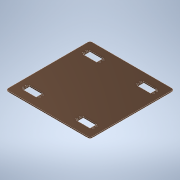
# Autodesk Inventor part: RobotBase
Saved by Autodesk Inventor 2022.3 (Build 263350000, 350)
## iProperties
Created: 2022-04-28
Part Number: RobotBase
Material: Bronze, Cast
Document SubType Name: Modeling
Designer: Robert Nies
Density: 8.87 g/cm^3
Appearance: Bronze - Satin
Author: Robert Nies
Autodesk Inventor part; units mm, degrees
ref_plane "YZ Plane" through (0, 0, 0) normal (1, 0, 0) x (0, 1, 0)
ref_plane "XZ Plane" through (0, 0, 0) normal (0, 1, 0) x (-1, 0, 0)
ref_plane "XY Plane" through (0, 0, 0) normal (0, 0, 1) x (1, 0, 0)
sketch "Sketch1" plane through (0, 0, 0) normal (0, 1, 0) x (-1, 0, 0)
  line L0 (0, 0) -> (-254, 0)
  line L1 (-254, 0) -> (-254, -254)
  line L2 (-254, -254) -> (0, -254)
  line L3 (0, -254) -> (0, 0)
  dimension "d0" = 254
  dimension "d1" = 254
  constraints: 8 end point, 2 parallel, 1 horizontal, 1 perpendicular
  measures "d0" distance of L2.end L1.end
  measures "d1" distance of L1.end L0.end
extrude "Extrusion1" add sketch "Sketch1" along normal blind 3.175
fillet "Fillet1" radius 6.35 4 edges at (0, 1.5875, 0) (254, 1.5875, 0) (254, 1.5875, -254) (0, 1.5875, -254)
sketch "Sketch2" plane through (0, 3.175, 0) normal (0, 1, 0) x (1, 0, 0)
  line L0 (247.65, 254) -> (6.35, 254) projected
  line L1 (0, 247.65) -> (0, 6.35) projected
  line L2 (25.4, 45.72) -> (66.04, 45.72)
  line L3 (66.04, 45.72) -> (66.04, 25.4)
  line L4 (66.04, 25.4) -> (25.4, 25.4)
  line L5 (25.4, 25.4) -> (25.4, 45.72)
  line L6 (254, 6.35) -> (254, 247.65) projected
  line L7 (6.35, 0) -> (247.65, 0) projected
  circle A0 centre (20.955, 30.635) radius 2.1828
  circle A1 centre (20.955, 40.485) radius 2.1828
  circle A2 centre (70.485, 40.485) radius 2.1828
  circle A3 centre (70.485, 30.635) radius 2.1828
  line L8 (25.4, 228.6) -> (66.04, 228.6)
  line L9 (66.04, 228.6) -> (66.04, 208.28)
  line L10 (66.04, 208.28) -> (25.4, 208.28)
  line L11 (25.4, 208.28) -> (25.4, 228.6)
  circle A4 centre (20.955, 213.515) radius 2.1828
  circle A5 centre (20.955, 223.365) radius 2.1828
  circle A6 centre (70.485, 223.365) radius 2.1828
  circle A7 centre (70.485, 213.515) radius 2.1828
  circle A8 centre (233.045, 223.365) radius 2.1828
  circle A9 centre (233.045, 213.515) radius 2.1828
  line L12 (228.6, 228.6) -> (228.6, 208.28)
  line L13 (187.96, 228.6) -> (228.6, 228.6)
  line L14 (228.6, 208.28) -> (187.96, 208.28)
  line L15 (187.96, 208.28) -> (187.96, 228.6)
  circle A10 centre (183.515, 223.365) radius 2.1828
  circle A11 centre (183.515, 213.515) radius 2.1828
  circle A12 centre (233.045, 40.485) radius 2.1828
  circle A13 centre (233.045, 30.635) radius 2.1828
  line L16 (228.6, 45.72) -> (228.6, 25.4)
  line L17 (187.96, 45.72) -> (228.6, 45.72)
  line L18 (228.6, 25.4) -> (187.96, 25.4)
  line L19 (187.96, 25.4) -> (187.96, 45.72)
  circle A14 centre (183.515, 40.485) radius 2.1828
  circle A15 centre (183.515, 30.635) radius 2.1828
  point P0 (0, 0)
  point P1 (45.72, 25.4)
  point P2 (25.4, 35.56)
  point P3 (45.72, 208.28)
  point P4 (25.4, 218.44)
  point P5 (127, 254)
  point P6 (208.28, 208.28)
  point P7 (187.96, 218.44)
  point P8 (208.28, 25.4)
  point P9 (187.96, 35.56)
  point P10 (208.28, 228.6)
  dimension "d13" = 40.64
  dimension "d14" = 20.32
  dimension "d19" = 25.4
  dimension "d20" = 25.4
  dimension "d23" = 4.3656
  dimension "d24" = 4.3656
  dimension "d25" = 4.3656
  dimension "d26" = 4.3656
  dimension "d27" = 9.85
  dimension "d28" = 9.85
  dimension "d29" = 49.53
  dimension "d30" = 49.53
  dimension "d31" = 0
  dimension "d32" = 0
  dimension "d33" = 4.445
  dimension "d34" = 5.235
  dimension "d35" = 40.64
  dimension "d36" = 20.32
  dimension "d37" = 4.3656
  dimension "d38" = 4.3656
  dimension "d39" = 4.3656
  dimension "d40" = 4.3656
  dimension "d41" = 9.85
  dimension "d42" = 9.85
  dimension "d43" = 49.53
  dimension "d44" = 49.53
  dimension "d45" = 0
  dimension "d46" = 0
  dimension "d47" = 4.445
  dimension "d48" = 5.235
  dimension "d51" = 25.4
  dimension "d52" = 25.4
  dimension "d53" = 40.64
  dimension "d54" = 20.32
  dimension "d55" = 4.3656
  dimension "d56" = 4.3656
  dimension "d57" = 4.3656
  dimension "d58" = 4.3656
  dimension "d59" = 9.85
  dimension "d60" = 9.85
  dimension "d61" = 49.53
  dimension "d62" = 49.53
  dimension "d63" = 0
  dimension "d64" = 0
  dimension "d65" = 4.445
  dimension "d66" = 5.235
  dimension "d69" = 40.64
  dimension "d70" = 20.32
  dimension "d71" = 4.3656
  dimension "d72" = 4.3656
  dimension "d73" = 4.3656
  dimension "d74" = 4.3656
  dimension "d75" = 9.85
  dimension "d76" = 9.85
  dimension "d77" = 49.53
  dimension "d78" = 49.53
  dimension "d79" = 0
  dimension "d80" = 0
  dimension "d81" = 4.445
  dimension "d82" = 5.235
  dimension "d85" = 25.4
  dimension "d86" = 25.4
  dimension "d87" = 25.4
  dimension "d88" = 25.4
  constraints: 32 end point, 16 centre point, 10 midpoint, 8 parallel, 4 horizontal, 4 perpendicular
  measures "d13" distance of L3.end L4.end
  measures "d14" distance of L2.end L3.end
  measures "d19" distance from line of L7 point (45.72, 25.4)
  measures "d20" distance from line of L1 point (25.4, 35.56)
  measures "d23" diameter of A0
  measures "d24" diameter of A1
  measures "d25" diameter of A2
  measures "d26" diameter of A3
  measures "d27" distance of A1.centre A0.centre
  measures "d28" distance of A3.centre A2.centre
  measures "d29" distance of A3.centre A0.centre
  measures "d30" distance of A1.centre A2.centre
  measures "d31" horizontal distance of A1.centre A0.centre
  measures "d32" vertical distance of A1.centre A2.centre
  measures "d33" distance from line of L5 A1.centre
  measures "d34" distance from line of L4 A0.centre
  measures "d35" distance of L9.end L10.end
  measures "d36" distance of L9.start L9.end
  measures "d37" diameter of A4
  measures "d38" diameter of A5
  measures "d39" diameter of A6
  measures "d40" diameter of A7
  measures "d41" distance of A5.centre A4.centre
  measures "d42" distance of A7.centre A6.centre
  measures "d43" distance of A7.centre A4.centre
  measures "d44" distance of A5.centre A6.centre
  measures "d45" horizontal distance of A5.centre A4.centre
  measures "d46" vertical distance of A5.centre A6.centre
  measures "d47" distance from line of L11 A5.centre
  measures "d48" distance from line of L10 A4.centre
  measures "d51" distance from line of point (127, 254) L8
  measures "d52" distance between parallel lines of L1 L11
  measures "d53" distance of L12.end L14.end
  measures "d54" distance of L12.start L12.end
  measures "d55" diameter of A11
  measures "d56" diameter of A10
  measures "d57" diameter of A8
  measures "d58" diameter of A9
  measures "d59" distance of A10.centre A11.centre
  measures "d60" distance of A9.centre A8.centre
  measures "d61" distance of A9.centre A11.centre
  measures "d62" distance of A10.centre A8.centre
  measures "d63" horizontal distance of A10.centre A11.centre
  measures "d64" vertical distance of A10.centre A8.centre
  measures "d65" distance from line of L15 A10.centre
  measures "d66" distance from line of L14 A11.centre
  measures "d69" distance of L16.end L18.end
  measures "d70" distance of L16.start L16.end
  measures "d71" diameter of A15
  measures "d72" diameter of A14
  measures "d73" diameter of A12
  measures "d74" diameter of A13
  measures "d75" distance of A14.centre A15.centre
  measures "d76" distance of A13.centre A12.centre
  measures "d77" distance of A13.centre A15.centre
  measures "d78" distance of A14.centre A12.centre
  measures "d79" horizontal distance of A14.centre A15.centre
  measures "d80" vertical distance of A14.centre A12.centre
  measures "d81" distance from line of L19 A14.centre
  measures "d82" distance from line of L18 A15.centre
  measures "d85" distance between parallel lines of L6 L12
  measures "d86" distance from line of L0 point (208.28, 228.6)
  measures "d87" distance between parallel lines of L7 L18
  measures "d88" distance between parallel lines of L6 L16
extrude "Extrusion2" cut sketch "Sketch2" against normal blind 3.175
equation "\"d13\" = d5"
equation "\"d14\" = d6"
equation "\"d20\" = d8"
equation "\"d28\" = d27"
equation "\"d29\" = d30"
equation "\"d33\" = -0.5 * d13 + 0.5 * d29"
equation "\"d34\" = -0.5 * d27 + 0.5 * d14"
equation "\"d35\" = d49"
equation "\"d36\" = d50"
equation "\"d42\" = d41"
equation "\"d43\" = d44"
equation "\"d47\" = -0.5 * d35 + 0.5 * d43"
equation "\"d48\" = -0.5 * d41 + 0.5 * d36"
equation "\"d53\" = d67"
equation "\"d54\" = d68"
equation "\"d60\" = d59"
equation "\"d61\" = d62"
equation "\"d65\" = -0.5 * d53 + 0.5 * d61"
equation "\"d66\" = -0.5 * d59 + 0.5 * d54"
equation "\"d69\" = d83"
equation "\"d70\" = d84"
equation "\"d76\" = d75"
equation "\"d77\" = d78"
equation "\"d81\" = -0.5 * d69 + 0.5 * d77"
equation "\"d82\" = -0.5 * d75 + 0.5 * d70"
equation "\"d5\" = 40.64"
equation "\"d6\" = 20.32"
equation "\"d49\" = 40.64"
equation "\"d50\" = 20.32"
equation "\"d67\" = 40.64"
equation "\"d68\" = 20.32"
equation "\"d83\" = 40.64"
equation "\"d84\" = 20.32"
equation "\"d8\" = 25.4"
body "Solid1"
